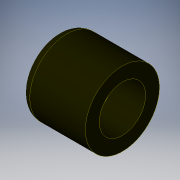
# Autodesk Inventor part: URLM8_p
Saved by Autodesk Inventor 2019 (Build 230136000, 136)
## iProperties
Created: 2024-01-11
Part Number: URLM8_p
Material: Generic
Catalog Web Link: www.cadenas.de
Description: URLH, URLM, URLL_p-Urethane Pushers -Tapped - Flat
Vendor: MISUMI
Document SubType Name: Modeling
Designer: psAdmin
Manufacturer: MISUMI
Mass: 0.265216 g
Surface Area: 3.25411 cm^2
Volume: 0.265216 cm^3
Density: 1 g/cm^3
Appearance: PSOLRGB-128-128-0
Category: PARTsolutions
Company: MISUMI
Title: URLM8
Author: Cadenas PARTsolutions
Comments: Urethane Pushers -Tapped - Flat
PSOL_IDENT_0: {$CADENAS_DATA/23d-libs/misumi/metric/34_cylinders/urlh_pusher.prj},175 {VTYP=3D},{NB=URLM8_p},{LINA=
PSOL_IDENT_1: URLM8},{NN=URLH, URLM, URLL_p},{DATE=04.06.2021 00:06:22},{GEOMDATE=17.02.2014 00:00:00},{VERSION=},
PSOL_IDENT_2: {LINEID=10},{WBVAR=MATP,HARD,M},{WBNUMERIC=}  {NB=URLM8_p},{LINA=URLM8},{KT=DUMMY},{PN=URLM8},{TYPE=
PSOL_IDENT_3: URLM},{MATCR=304 Stainless Steel},{MATP=2},{MATP1='1', 'Ether Type Polyurethane', '2', 'Ester Type P
PSOL_IDENT_4: olyurethane'},{HARD=2},{HARD0='2', 'Shore A70','3','Shore A50'},{D=8},{L=12},{M=1},{MALG='1','M3x0.5'
PSOL_IDENT_5: },{SR1=8},{R2=1.0},{LL1=5},{LL2=4},{W=7},{NDM=5},{P=0.50},{ALG=},{CRC=1},{CR1=9.5}
NB: URLM8_p
NN: URLH, URLM, URLL_p
NT: Urethane Pushers -Tapped - Flat
NBSYN: $PN._p
LINA: URLM8
CATALOG: Misumi
PN: URLM8
MATCR: 304 Stainless Steel
MATP: Ester Type Polyurethane
HARD: Shore A70
D: 8
L: 12
M: M3x0.5
SR1: 8
R2: 1
LL1: 5
LL2: 4
W: 7
SUPPLIER: MISUMI
ARTICLENO: URLM8_p
BOMINFO: URLM8
CREATOR: CADENAS GmbH
Autodesk Inventor part; units mm, degrees
sketch "Sketch_1" plane through (0, 0, 0) normal (0, 0, 1) x (1, 0, 0)
  line L0 (12, 0) -> (0, 0)
  line L1 (0, 0) -> (0, 3)
  arc A0 (1, 4) -> (0, 3) centre (1, 3) ccw
  line L2 (1, 4) -> (7, 4)
  line L3 (7, 4) -> (7, 2.5)
  line L4 (7, 2.5) -> (3.5, 2.5)
  line L5 (3.5, 2.5) -> (2.5, 1.5)
  line L6 (2.5, 1.5) -> (2.5, 0)
  line L7 (2.5, 0) -> (0, 0)
  constraints: 16 end point, 2 point on circle, 1 centre point
revolve "Revolution1" add sketch "Sketch_1" angle 360 about axis through (12, 0, 0) along (1, 0, 0)
ref_plane "pusher_XY" through (7, 0, 0) normal (1, 0, 0) x (0, 0, -1)
ref_plane "pusher_YZ" through (7, 0, 0) normal (0, 0, -1) x (0, 1, 0)
ref_plane "pusher_ZX" through (7, 0, 0) normal (0, 1, 0) x (1, 0, 0)
body "Solid1"
